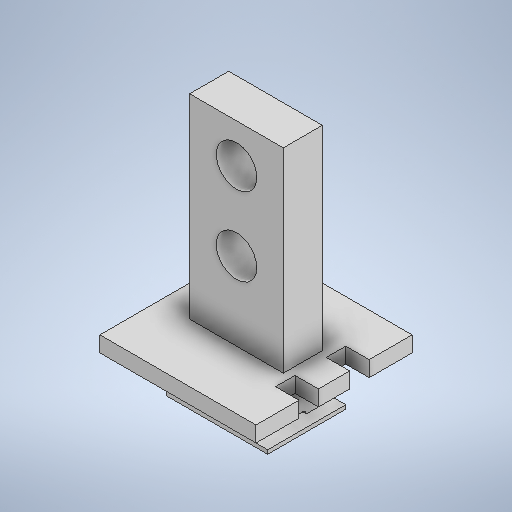
# Autodesk Inventor part: 單線圈感測器上
Saved by Autodesk Inventor 2025.2 (Build 292293000, 293)
## iProperties
Created: 2025-06-16
Part Number: 單線圈感測器上
Material: 一般
Document SubType Name: Modeling
Designer: 123
Density: 1 g/cm^3
Appearance: 預設
Author: 123
Autodesk Inventor part; units mm, degrees
ref_plane "YZ Plane" through (0, 0, 0) normal (1, 0, 0) x (0, 1, 0)
ref_plane "XZ Plane" through (0, 0, 0) normal (0, 1, 0) x (-1, 0, 0)
ref_plane "XY Plane" through (0, 0, 0) normal (0, 0, 1) x (1, 0, 0)
sketch "草圖1" plane through (0, 0, 0) normal (0, 0, 1) x (1, 0, 0)
  point P0 (0, 0)
sketch "草圖2" plane through (0, 0, 0) normal (0, 1, 0) x (-1, 0, 0)
  line L0 (6, 2.5) -> (-6, 2.5)
  line L1 (-6, 2.5) -> (-6, -2.5)
  line L2 (-6, -2.5) -> (6, -2.5)
  line L3 (6, -2.5) -> (6, 2.5)
  line L4 (6, 2.5) -> (-6, -2.5) construction
  line L5 (-6, 2.5) -> (6, -2.5) construction
  point P0 (0, 0)
  dimension "d0" = 5
  dimension "d1" = 12
  constraints: 12 end point, 2 midpoint, 2 parallel, 1 horizontal, 1 perpendicular
  measures "d0" distance of L2.end L0.start
  measures "d1" distance of L0.start L0.end
extrude "擠出1" add sketch "草圖2" along normal blind 25
sketch "草圖3" plane through (-6, 0, 2.5) normal (0, 0, 1) x (1, 0, 0)
  circle A0 centre (6, 10) radius 2.6
  circle A1 centre (6, 20) radius 2.6
  line L0 (0, 0) -> (12, 0) projected
  point P0 (6, 0)
  point P1 (6, 0)
  dimension "d4" = 5.2
  dimension "d5" = 5.2
  dimension "d6" = 10
  dimension "d7" = 10
  constraints: 2 centre point, 1 midpoint
  measures "d4" diameter of A0
  measures "d5" diameter of A1
  measures "d6" distance of point (6, 0) A0.centre
  measures "d7" distance of A0.centre A1.centre
extrude "擠出2" cut sketch "草圖3" against normal blind 5.2
sketch "草圖4" plane through (0, 0, 0) normal (0, -1, 0) x (1, 0, 0)
  line L0 (-10, -10) -> (10, -10)
  line L1 (10, -10) -> (10, 10)
  line L2 (10, 10) -> (-10, 10)
  line L3 (-10, 10) -> (-10, -10)
  line L4 (-10, -10) -> (10, 10) construction
  line L5 (10, -10) -> (-10, 10) construction
  point P0 (0, 0)
  dimension "d10" = 20
  dimension "d11" = 20
  constraints: 12 end point, 2 midpoint, 2 parallel, 1 horizontal, 1 perpendicular
  measures "d10" distance of L0.end L1.end
  measures "d11" distance of L0.start L0.end
extrude "擠出3" add sketch "草圖4" along normal blind 2
sketch "草圖5" plane through (0, -2, 0) normal (0, -1, 0) x (1, 0, 0)
  line L0 (-0.95, -1.15) -> (0.95, -1.15)
  line L1 (0.95, -1.15) -> (0.95, 1.15)
  line L2 (0.95, 1.15) -> (-0.95, 1.15)
  line L3 (-0.95, 1.15) -> (-0.95, -1.15)
  line L4 (-0.95, -1.15) -> (0.95, 1.15) construction
  line L5 (0.95, -1.15) -> (-0.95, 1.15) construction
  point P0 (0, 0)
  dimension "d14" = 1.9
  dimension "d15" = 2.3
  constraints: 12 end point, 2 midpoint, 2 parallel, 1 horizontal, 1 perpendicular
  measures "d14" distance of L1.end L2.end
  measures "d15" distance of L2.end L0.start
extrude "擠出4" add sketch "草圖5" along normal blind 5
sketch "草圖6" plane through (0, -2, 0) normal (0, -1, 0) x (1, 0, 0)
  line L0 (-4, -3) -> (4, -3)
  line L1 (4, -3) -> (4, 3)
  line L2 (4, 3) -> (-4, 3)
  line L3 (-4, 3) -> (-4, -3)
  line L4 (-4, -3) -> (4, 3) construction
  line L5 (4, -3) -> (-4, 3) construction
  line L6 (-5, -3.75) -> (5, -3.75)
  line L7 (5, -3.75) -> (5, 3.75)
  line L8 (5, 3.75) -> (-5, 3.75)
  line L9 (-5, 3.75) -> (-5, -3.75)
  line L10 (-5, -3.75) -> (5, 3.75) construction
  line L11 (5, -3.75) -> (-5, 3.75) construction
  point P0 (0, 0)
  dimension "d18" = 6
  dimension "d19" = 8
  dimension "d20" = 10
  constraints: 24 end point, 4 midpoint, 4 parallel, 2 horizontal, 2 perpendicular, 1 point on line
  measures "d18" distance of L0.end L1.end
  measures "d19" distance of L1.end L2.end
  measures "d20" distance of L7.end L8.end
extrude "擠出5" add sketch "草圖6" along normal blind 5
sketch "草圖7" plane through (5, -2, 3.75) normal (1, 0, 0) x (0, 0, -1)
  line L0 (7.5, -5) -> (0, -5) projected
  line L1 (2.3009, -5) -> (5.1991, -5) construction
  line L2 (2.75, -4.5509) -> (4.75, -4.5509)
  line L3 (4.75, -5.4491) -> (2.75, -5.4491)
  arc A0 (2.75, -4.5509) -> (2.75, -5.4491) centre (2.75, -5) ccw
  arc A1 (4.75, -5.4491) -> (4.75, -4.5509) centre (4.75, -5) ccw
  line L4 (-6.25, 0) -> (13.75, 0) projected
  line L5 (3.75, 0) -> (3.75, -5)
  line L6 (0, 0) -> (0, -5) projected
  point P0 (3.75, 2)
  point P1 (5.1991, -5)
  dimension "d23" = 2
  dimension "d26" = 3.75
  constraints: 10 end point, 6 point on circle, 4 point on line, 4 tangent, 2 centre point, 2 midpoint, 1 parallel, 1 perpendicular
  measures "d23" distance of L3.end L3.start
  measures "d26" distance between parallel lines of L6 L5
extrude "擠出6" cut sketch "草圖7" against normal blind 2 contours L0 L5 L2 A1 | L0 A0 L2 L5
sketch "草圖8" plane through (0, 0, 0) normal (0, 1, 0) x (1, 0, 0)
  line L0 (10, 10) -> (10, -10) projected
  line L1 (7, -4.5) -> (10, -4.5)
  line L2 (10, -4.5) -> (10, -2)
  line L3 (10, -2) -> (7, -2)
  line L4 (7, -2) -> (7, -4.5)
  line L5 (7, 2) -> (10, 2)
  line L6 (10, 2) -> (10, 4.5)
  line L7 (10, 4.5) -> (7, 4.5)
  line L8 (7, 4.5) -> (7, 2)
  point P0 (0, 0)
  point P1 (10, 0)
  point P2 (10, 0)
  dimension "d27" = 3
  dimension "d28" = 2.5
  dimension "d29" = 2.5
  dimension "d30" = 2
  dimension "d31" = 2
  constraints: 16 end point, 4 parallel, 3 point on line, 2 horizontal, 2 midpoint, 2 perpendicular
  measures "d27" distance of L1.start L1.end
  measures "d28" distance of L3.end L1.start
  measures "d29" distance of L7.end L5.start
  measures "d30" distance from line of point (10, 0) L3
  measures "d31" distance from line of point (10, 0) L5
extrude "擠出7" cut sketch "草圖8" against normal blind 2
sketch "草圖9" plane through (0, -7, 0) normal (0, -1, 0) x (1, 0, 0)
  line L0 (6.5, 5) -> (-6.5, 5)
  line L1 (-6.5, 5) -> (-6.5, -5)
  line L2 (-6.5, -5) -> (6.5, -5)
  line L3 (6.5, -5) -> (6.5, 5)
  line L4 (6.5, 5) -> (-6.5, -5) construction
  line L5 (-6.5, 5) -> (6.5, -5) construction
  point P0 (0, 0)
  dimension "d34" = 10
  dimension "d35" = 13
  constraints: 12 end point, 2 midpoint, 2 parallel, 1 horizontal, 1 perpendicular
  measures "d34" distance of L2.end L0.start
  measures "d35" distance of L1.end L2.end
extrude "擠出8" add sketch "草圖9" along normal blind 0.5
sketch "草圖10" plane through (0, -7.5, 0) normal (0, -1, 0) x (1, 0, 0)
  line L0 (-4, 3) -> (-4, -3) projected
  line L1 (4, 3) -> (-4, 3)
  line L2 (-4, 3) -> (-4, -3)
  line L3 (-4, -3) -> (4, -3)
  line L4 (4, -3) -> (4, 3)
  line L5 (4, 3) -> (-4, -3) construction
  line L6 (-4, 3) -> (4, -3) construction
  point P0 (0, 0)
  constraints: 12 end point, 2 midpoint, 2 parallel, 1 horizontal, 1 perpendicular
extrude "擠出9" cut sketch "草圖10" against normal blind 5
sketch "草圖11" plane through (0, -2.5, 0) normal (0, -1, 0) x (1, 0, 0)
  line L0 (0.95, -1.15) -> (-0.95, -1.15) projected
  line L1 (0.95, 1.15) -> (-0.95, 1.15)
  line L2 (-0.95, 1.15) -> (-0.95, -1.15)
  line L3 (-0.95, -1.15) -> (0.95, -1.15)
  line L4 (0.95, -1.15) -> (0.95, 1.15)
  line L5 (0.95, 1.15) -> (-0.95, -1.15) construction
  line L6 (-0.95, 1.15) -> (0.95, -1.15) construction
  point P0 (0, 0)
  constraints: 12 end point, 2 midpoint, 2 parallel, 1 horizontal, 1 perpendicular
extrude "擠出10" add sketch "草圖11" along normal blind 5
equation "\"d8\" = d5"
